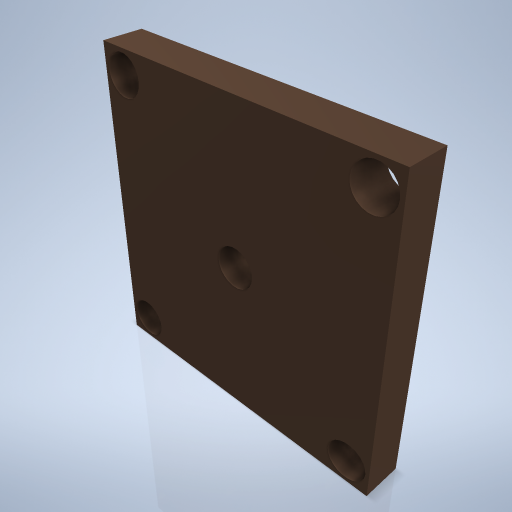
# Autodesk Inventor part: cylinder_lid
Saved by Autodesk Inventor 2024.2 (Build 282272000, 272)
## iProperties
Created: 2024-05-14
Part Number: cylinder_lid
Material: Bronze, Guss
Document SubType Name: Modeling
Designer: Fabri
Density: 8.87 g/cm^3
Appearance: Bronze - satiniert
Author: Fabri
Autodesk Inventor part; units mm, degrees
ref_plane "YZ Plane" through (0, 0, 0) normal (1, 0, 0) x (0, 1, 0)
ref_plane "XZ Plane" through (0, 0, 0) normal (0, 1, 0) x (-1, 0, 0)
ref_plane "XY Plane" through (0, 0, 0) normal (0, 0, 1) x (1, 0, 0)
sketch "Skizze1" plane through (0, 0, 0) normal (0, 1, 0) x (-1, 0, 0)
  line L0 (-25, 25) -> (25, 25)
  line L1 (25, 25) -> (25, -25)
  line L2 (25, -25) -> (-25, -25)
  line L3 (-25, -25) -> (-25, 25)
  line L4 (-25, 25) -> (25, -25) construction
  line L5 (25, 25) -> (-25, -25) construction
  point P0 (0, 0)
  dimension "d0" = 50
  dimension "d1" = 50
  constraints: 12 end point, 2 midpoint, 2 parallel, 1 horizontal, 1 perpendicular
  measures "d0" distance of L1.end L2.end
  measures "d1" distance of L0.end L1.end
extrude "Extrusion1" add sketch "Skizze1" along normal blind 6.5
sketch "Skizze2" plane through (0, 6.5, 0) normal (0, 1, 0) x (1, 0, 0)
  circle A0 centre (0, 0) radius 13.5
  dimension "d4" = 27
  constraints: 1 centre point, 1 coincident
  measures "d4" diameter of A0
extrude "Extrusion2" add sketch "Skizze2" along normal blind 1.5
sketch "Skizze3" plane through (0, 8, 0) normal (0, 1, 0) x (1, 0, 0)
  circle A0 centre (0, 0) radius 13.5 projected
  constraints: 1 coincident
hole "Bohrung1" at (0, 8, 0) direction (0, -1, 0) diameter 6.5 depth 8
sketch "Skizze4" plane through (0, 6.5, 0) normal (0, 1, 0) x (1, 0, 0)
  line L0 (25, -25) -> (25, 25) projected
  line L1 (25, 0) -> (-25, 0) construction
  line L2 (-25, 25) -> (-25, -25) projected
  line L3 (-25, -25) -> (25, -25) projected
  line L4 (0, -25) -> (0, 25) construction
  line L5 (25, 25) -> (-25, 25) projected
  point P0 (0, 0)
  point P1 (-21.124, 21.124)
  point P2 (-21.124, -21.124)
  point P3 (21.124, -21.124)
  point P4 (21.124, 21.124)
  dimension "d29" = 42.248
  constraints: 4 end point, 4 midpoint, 4 symmetric about line, 2 horizontal alignment, 2 vertical alignment
  measures "d29" distance of point (-21.124, -21.124) point (21.124, -21.124)
hole "Bohrung2" at (-21.124, 6.5, -21.124) at (-21.124, 6.5, 21.124) at (21.124, 6.5, 21.124) at (21.124, 6.5, -21.124) direction (0, -1, 0) diameter 6.5 depth 6.5
